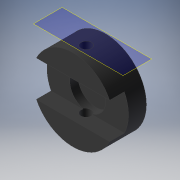
# Autodesk Inventor part: Part2
Saved by Autodesk Inventor 2019 (Build 230136000, 136)
## iProperties
Created: 2020-01-30
Part Number: Part2
Material: Generic
Document SubType Name: Modeling
Designer: marsikovabarbora
Density: 1 g/cm^3
Appearance: Default
Author: marsikovabarbora
Autodesk Inventor part; units mm, degrees
ref_plane "YZ Plane" through (0, 0, 0) normal (1, 0, 0) x (0, 1, 0)
ref_plane "XZ Plane" through (0, 0, 0) normal (0, 1, 0) x (-1, 0, 0)
ref_plane "XY Plane" through (0, 0, 0) normal (0, 0, 1) x (1, 0, 0)
sketch "Sketch1" plane through (0, 0, 0) normal (0, 0, 1) x (1, 0, 0)
  line L0 (-17.5, 0) -> (17.5, 0) construction
  line L1 (0, -17.5) -> (0, 17.5) construction
  circle A0 centre (0, 0) radius 12.5
  dimension "d0" = 25
  constraints: 1 centre point, 1 coincident
  measures "d0" diameter of A0
extrude "Extrusion1" add sketch "Sketch1" along normal blind 10
sketch "Sketch2" plane through (0, 0, 10) normal (0, 0, 1) x (1, 0, 0)
  circle A0 centre (0, 0) radius 12.5 construction
  circle A1 centre (0, 0) radius 5.5
  dimension "d3" = 11
  constraints: 1 centre point, 1 coincident
  measures "d3" diameter of A1
extrude "Extrusion2" cut sketch "Sketch2" against normal blind 7
sketch "Sketch3" plane through (0, 0, 10) normal (0, 0, 1) x (1, 0, 0)
  circle A0 centre (0, 0) radius 5.5 projected
  circle A1 centre (0, 0) radius 12.5 construction
  line L0 (13.9889, -5.5) -> (-13.9889, -5.5)
  line L1 (-13.9889, -5.5) -> (-13.9889, 5.5)
  line L2 (-13.9889, 5.5) -> (13.9889, 5.5)
  line L3 (13.9889, 5.5) -> (13.9889, -5.5)
  line L4 (13.9889, -5.5) -> (-13.9889, 5.5) construction
  line L5 (-13.9889, -5.5) -> (13.9889, 5.5) construction
  circle A2 centre (0, 0) radius 5.5 construction
  constraints: 12 end point, 2 midpoint, 2 parallel, 1 horizontal, 1 perpendicular, 1 tangent
extrude "Extrusion3" cut sketch "Sketch3" against normal blind 4.5 contours A0 L2 L3 L0 | A0 L0 L1 L2
ref_plane "Work Plane1" through (0, 12.5, 0) normal (0, -1, 0) x (1, 0, 0)
sketch "Sketch4" plane through (0, 12.5, 0) normal (0, -1, 0) x (1, 0, 0)
  line L0 (-12.5, 0) -> (12.5, 0) construction
  line L1 (-11.225, 10) -> (-11.225, 5.5) construction
  line L2 (-11.225, 5.5) -> (-11.225, 5.5) construction
  line L3 (-11.225, 5.5) -> (-11.225, 10) construction
  line L4 (11.225, 10) -> (-11.225, 10) construction
  line L5 (11.225, 10) -> (11.225, 5.5) construction
  line L6 (11.225, 5.5) -> (11.225, 5.5) construction
  line L7 (11.225, 5.5) -> (11.225, 10) construction
  line L8 (-11.225, 10) -> (11.225, 10) construction
  line L9 (0, -2) -> (0, 12) construction
  circle A0 centre (0, 6) radius 1.6
  point P0 (0, 0)
  dimension "d8" = 3.2
  dimension "d9" = 4
  constraints: 1 centre point, 1 point on line
  measures "d8" diameter of A0
  measures "d9" distance from line of L4 A0.centre
extrude "Extrusion4" cut sketch "Sketch4" along normal through all
body "Solid1"
